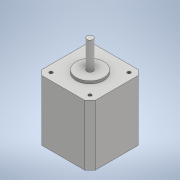
# Autodesk Inventor part: ステッピングモータ
Saved by Autodesk Inventor 2020 (Build 240168000, 168)
## iProperties
Created: 2020-06-19
Part Number: ステッピングモータ
Material: 一般
Document SubType Name: Modeling
Designer: bsat3
Density: 1 g/cm^3
Appearance: 既定
Author: bsat3
Autodesk Inventor part; units mm, degrees
ref_plane "YZ Plane" through (0, 0, 0) normal (1, 0, 0) x (0, 1, 0)
ref_plane "XZ Plane" through (0, 0, 0) normal (0, 1, 0) x (-1, 0, 0)
ref_plane "XY Plane" through (0, 0, 0) normal (0, 0, 1) x (1, 0, 0)
sketch "スケッチ1" plane through (0, 0, 0) normal (0, 0, 1) x (1, 0, 0)
  line L0 (16.9587, -21.15) -> (-16.9587, -21.15)
  line L1 (-21.15, -16.9587) -> (-21.15, 16.9587)
  line L2 (-16.9587, 21.15) -> (16.9587, 21.15)
  line L3 (21.15, 16.9587) -> (21.15, -16.9587)
  line L4 (21.15, -21.15) -> (-21.15, 21.15) construction
  line L5 (-21.15, -21.15) -> (21.15, 21.15) construction
  line L6 (-16.9587, 21.15) -> (-21.15, 16.9587)
  line L7 (-21.15, -16.9587) -> (-16.9587, -21.15)
  line L8 (16.9587, -21.15) -> (21.15, -16.9587)
  line L9 (21.15, 16.9587) -> (16.9587, 21.15)
  point P0 (0, 0)
  dimension "d4" = 360
  dimension "d0" = 42.3
  dimension "d1" = 42.3
  constraints: 20 end point, 2 midpoint, 2 parallel, 2 perpendicular, 1 horizontal, 13 other
  measures "d0" distance of L4.end L5.end
  measures "d1" distance of L5.end L4.start
extrude "押し出し1" add sketch "スケッチ1" along normal blind 48
sketch "スケッチ2" plane through (0, 0, 48) normal (0, 0, 1) x (1, 0, 0)
  line L0 (15.5, -15.5) -> (-15.5, -15.5)
  line L1 (-15.5, -15.5) -> (-15.5, 15.5)
  line L2 (-15.5, 15.5) -> (15.5, 15.5)
  line L3 (15.5, 15.5) -> (15.5, -15.5)
  line L4 (15.5, -15.5) -> (-15.5, 15.5) construction
  line L5 (-15.5, -15.5) -> (15.5, 15.5) construction
  point P0 (0, 0)
  point P1 (15.5, 15.5)
  dimension "d8" = 31
  dimension "d9" = 31
  constraints: 12 end point, 4 coincident, 2 midpoint, 2 parallel, 1 horizontal, 1 perpendicular
  measures "d8" distance of L2.end L0.start
  measures "d9" distance of L1.end L2.end
hole "穴1" at (-15.5, 15.5, 48) at (15.5, 15.5, 48) at (15.5, -15.5, 48) at (-15.5, -15.5, 48) direction (0, 0, -1) diameter 2.459 depth 4.5 thread size "M3x0.5" class "6H" standard "ISO Metric profile"
sketch "スケッチ3" plane through (0, 0, 48) normal (0, 0, 1) x (1, 0, 0)
  circle A0 centre (0, 0) radius 11
  dimension "d17" = 22
  constraints: 1 centre point, 1 coincident
  measures "d17" diameter of A0
extrude "押し出し2" add sketch "スケッチ3" along normal blind 2
sketch "スケッチ4" plane through (0, 0, 50) normal (0, 0, 1) x (1, 0, 0)
  circle A0 centre (0, 0) radius 2.5
  dimension "d20" = 5
  constraints: 1 centre point, 1 coincident
  measures "d20" diameter of A0
extrude "押し出し3" add sketch "スケッチ4" along normal blind 22
